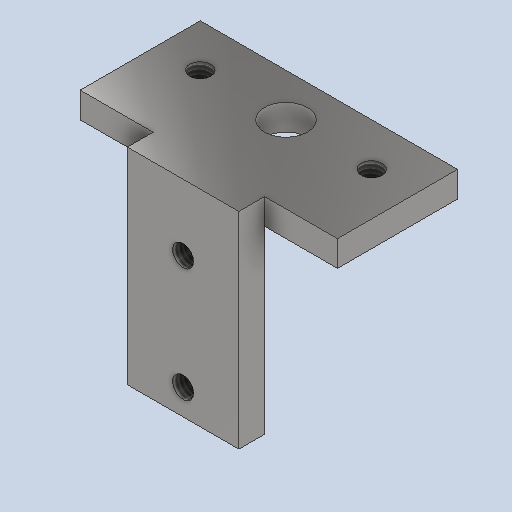
# Autodesk Inventor part: adapter
Saved by Autodesk Inventor 2022.1 (Build 261234020, 234B)
## iProperties
Created: 2022-05-02
Part Number: adapter
Material: Stal nierdzewna 440C
Document SubType Name: Modeling
Designer: Kacper Kaczmarski
Density: 7.75 g/cm^3
Appearance: Częściowo polerowany
Mass: 16.1208 g
Surface Area: 19.3456 cm^2
Volume: 2.08011 cm^3
Author: Kacper Kaczmarski
Autodesk Inventor part; units mm, degrees
ref_plane "YZ Plane" through (0, 0, 0) normal (1, 0, 0) x (0, 1, 0)
ref_plane "XZ Plane" through (0, 0, 0) normal (0, 1, 0) x (-1, 0, 0)
ref_plane "XY Plane" through (0, 0, 0) normal (0, 0, 1) x (1, 0, 0)
sketch "Szkic1" plane through (0, 0, 0) normal (0, 0, 1) x (1, 0, 0)
  line L0 (-9.1, 0) -> (9.1, 0) projected
  line L1 (0, -4.8) -> (0, 28.8) projected
  line L2 (-6.5, 24) -> (6.5, 24)
  line L3 (6.5, 24) -> (6.5, 0)
  line L4 (6.5, 0) -> (-6.5, 0)
  line L5 (-6.5, 0) -> (-6.5, 24)
  line L6 (0, 24) -> (0, 0)
  dimension "d0" = 13
  dimension "d1" = 24
  constraints: 10 end point, 2 parallel, 1 collinear, 1 horizontal, 1 midpoint, 1 perpendicular, 2 other
  measures "d0" distance of L3.end L4.end
  measures "d1" distance of L2.end L3.end
extrude "Wyciągnięcie proste1" add sketch "Szkic1" against normal blind 17
sketch "Szkic2" plane through (6.5, 0, 0) normal (1, 0, 0) x (0, 0, -1)
  line L0 (17, 24) -> (17, 0) projected
  line L1 (17, 0) -> (3, 0)
  line L2 (3, 0) -> (3, 21)
  line L3 (3, 21) -> (17, 21)
  line L4 (17, 21) -> (17, 0)
  point P0 (0, 0)
  dimension "d4" = 14
  dimension "d5" = 21
  constraints: 8 end point, 2 parallel, 1 horizontal, 1 perpendicular
  measures "d4" distance of L2.end L3.end
  measures "d5" distance of L1.end L2.end
extrude "Wyciągnięcie proste2" cut sketch "Szkic2" against normal blind 13
sketch "Szkic3" plane through (0, 0, 0) normal (0, 0, 1) x (1, 0, 0)
  line L0 (6.5, 24) -> (-6.5, 24) projected
  line L1 (-6.5, 0) -> (6.5, 0) projected
  point P0 (0, 0)
  point P1 (0, 16.3)
  point P2 (0, 3)
  dimension "d8" = 7.7
  dimension "d10" = 3
  measures "d8" distance from line of L0 point (0, 16.3)
  measures "d10" distance from line of L1 point (0, 3)
hole "Otwór1" at (0, 16.3, 0) at (0, 3, 0) direction (0, 0, -1) diameter 2.459 end through all thread size "M3x0.5" class "6H" standard "ISO Metric profile"
sketch "Szkic4" plane through (-6.5, 24, 0) normal (0, 1, 0) x (1, 0, 0)
  line L0 (13, 3) -> (0, 3) projected
  line L1 (0, 17) -> (13, 17) projected
  line L2 (6.5, 17) -> (6.5, 3)
  circle A0 centre (6.5, 12) radius 2.5
  line L3 (13, 0) -> (13, 17) projected
  line L4 (19, 12) -> (-6, 12)
  line L5 (0, 3) -> (-6, 3)
  line L6 (-6, 3) -> (-6, 17)
  line L7 (-6, 17) -> (0, 17)
  line L8 (0, 17) -> (0, 3)
  line L9 (13, 3) -> (19, 3)
  line L10 (19, 3) -> (19, 17)
  line L11 (19, 17) -> (13, 17)
  line L12 (13, 17) -> (13, 3)
  line L13 (-3.5, 3) -> (-3.5, 17)
  line L14 (0, 0) -> (0, 17) projected
  line L15 (0, 3) -> (0, 17)
  line L16 (16.5, 3) -> (16.5, 17)
  point P0 (6.5, 0)
  point P1 (0, 12)
  dimension "d18" = 5
  dimension "d20" = 5
  dimension "d21" = 6
  dimension "d22" = 6
  dimension "d23" = 3.5
  constraints: 26 end point, 6 point on line, 4 parallel, 4 perpendicular, 3 midpoint, 2 horizontal, 2 symmetric about line, 1 centre point, 1 vertical
  measures "d18" diameter of A0
  measures "d20" distance between parallel lines of L1 L4
  measures "d21" distance of L6.end L7.end
  measures "d22" distance of L11.end L10.end
  measures "d23" distance between parallel lines of L13 L14
extrude "Wyciągnięcie proste3" add sketch "Szkic4" against normal blind 3 contours L3 L4 L16 L9 | L3 L11 L16 L4 | L16 L4 L10 L9 | L5 L13 L4 L8 | L16 L11 L10 L4 | L5 L6 L4 L13 | L4 L13 L7 L8 | L4 L6 L7 L13
sketch "Szkic5" plane through (-6.5, 24, 0) normal (0, 1, 0) x (1, 0, 0)
  line L0 (13, 3) -> (0, 3) projected
  line L1 (6.5, 0) -> (6.5, 17)
  line L2 (-6, 17) -> (19, 17) projected
  line L3 (19, 17) -> (19, 3) projected
  line L4 (19, 12) -> (-6.0034, 12)
  line L5 (19, 3) -> (13, 3) projected
  line L6 (16.5, 3) -> (16.5, 17)
  line L7 (-3.5, 3) -> (-3.5, 17)
  circle A0 centre (6.4983, 12) radius 2.5
  dimension "d4" = 14
  dimension "d5" = 21
  dimension "d26" = 5
  dimension "d27" = 2.5
  dimension "d28" = 5
  constraints: 8 end point, 3 point on line, 2 midpoint, 2 perpendicular, 2 symmetric about line, 1 centre point
  measures "d26" distance between parallel lines of L4 L2
  measures "d27" distance between parallel lines of L6 L3
  measures "d28" diameter of A0
extrude "Wyciągnięcie proste4" cut sketch "Szkic5" against normal blind 3 contours A0 L4 L1 | L1 L4 A0 | L4 A0 L1 | L1 A0 L4
sketch "Szkic6" plane through (-6.5, 24, 0) normal (0, 1, 0) x (1, 0, 0)
  line L0 (6.5, 0) -> (6.5, 17)
  line L1 (-6, 17) -> (19, 17) projected
  line L2 (19, 17) -> (19, 3) projected
  line L3 (19, 12) -> (-5.9544, 12)
  line L4 (19, 3) -> (13, 3) projected
  line L5 (16.5, 3) -> (16.5, 17)
  line L6 (-3.5, 3) -> (-3.5, 17)
  point P0 (16.5, 12)
  point P1 (-3.5, 12)
  dimension "d31" = 5
  dimension "d32" = 2.5
  constraints: 8 end point, 7 point on line, 2 perpendicular, 2 symmetric about line, 1 midpoint
  measures "d31" distance between parallel lines of L3 L1
  measures "d32" distance between parallel lines of L5 L2
hole "Otwór2" at (10, 24, -12) at (-10, 24, -12) direction (0, -1, 0) diameter 2.459 end through all thread size "M3x0.5" class "6H" standard "ISO Metric profile"
sketch "Szkic7" plane through (-6.5, 24, 0) normal (0, 1, 0) x (1, 0, 0)
  line L0 (19, 3) -> (13, 3) projected
  line L1 (19, 3) -> (21.5, 3)
  line L2 (21.5, 3) -> (21.5, 17)
  line L3 (21.5, 17) -> (19, 17)
  line L4 (19, 17) -> (19, 3)
  line L5 (-6, 3) -> (-6, 17) projected
  line L6 (-6, 3) -> (-8.5, 3)
  line L7 (-8.5, 3) -> (-8.5, 17)
  line L8 (-8.5, 17) -> (-6, 17)
  line L9 (-6, 17) -> (-6, 3)
  point P0 (6.5, 0)
  dimension "d40" = 2.5
  dimension "d41" = 2.5
  constraints: 16 end point, 4 parallel, 2 horizontal, 2 perpendicular, 1 point on line
  measures "d40" distance of L3.end L2.end
  measures "d41" distance of L7.end L8.end
extrude "Wyciągnięcie proste5" add sketch "Szkic7" against normal blind 3
